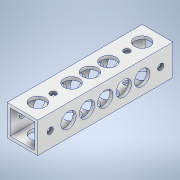
# Autodesk Inventor part: 前後直動12x12_3
Saved by Autodesk Inventor 2020.3 (Build 243373000, 373)
## iProperties
Created: 2020-07-05
Part Number: 前後直動12x12_3
Material: アルミニウム 6061
Document SubType Name: Modeling
Designer: totot
Density: 2.7 g/cm^3
Appearance: アルミニウム - フラット
Mass: 14.2052 g
Surface Area: 72.9 cm^2
Volume: 5.26118 cm^3
Author: totot
Autodesk Inventor part; units mm, degrees
ref_plane "YZ Plane" through (0, 0, 0) normal (1, 0, 0) x (0, 1, 0)
ref_plane "XZ Plane" through (0, 0, 0) normal (0, 1, 0) x (-1, 0, 0)
ref_plane "XY Plane" through (0, 0, 0) normal (0, 0, 1) x (1, 0, 0)
sketch "スケッチ1" plane through (0, 0, 0) normal (0, 0, 1) x (1, 0, 0)
  line L0 (0, 0) -> (-15, 0)
  line L1 (-15, 0) -> (-15, -15)
  line L2 (-15, -15) -> (0, -15)
  line L3 (0, -15) -> (0, 0)
  line L4 (-13.5, -1.5) -> (-1.5, -1.5)
  line L5 (-1.5, -1.5) -> (-1.5, -13.5)
  line L6 (-1.5, -13.5) -> (-13.5, -13.5)
  line L7 (-13.5, -13.5) -> (-13.5, -1.5)
  dimension "d0" = 15
  dimension "d1" = 15
  dimension "d2" = 12
  dimension "d3" = 12
  dimension "d4" = 1.5
  dimension "d5" = 1.5
  constraints: 16 end point, 4 parallel, 2 horizontal, 2 perpendicular
  measures "d0" distance of L2.end L1.end
  measures "d1" distance of L1.end L0.end
  measures "d2" distance of L5.end L6.end
  measures "d3" distance of L4.end L5.end
  measures "d4" distance between parallel lines of L1 L7
  measures "d5" distance between parallel lines of L4 L0
extrude "押し出し1" add sketch "スケッチ1" along normal blind 66
sketch "スケッチ2" plane through (0, -15, 0) normal (1, 0, 0) x (0, 0, -1)
  line L0 (0, 15) -> (-66, 15) projected
  line L1 (0, 0) -> (0, 15) projected
  line L2 (-66, 0) -> (-66, 15) projected
  point P0 (-60, 7.5)
  point P1 (-6, 7.5)
  dimension "d8" = 7.5
  dimension "d9" = 7.5
  dimension "d10" = 6
  dimension "d11" = 6
  measures "d8" distance from line of point (-60, 7.5) L0
  measures "d9" distance from line of point (-6, 7.5) L0
  measures "d10" distance from line of point (-6, 7.5) L1
  measures "d11" distance from line of point (-60, 7.5) L2
hole "穴1" at (0, -7.5, 60) at (0, -7.5, 6) direction (-1, 0, 0) diameter 3 end through all
sketch "スケッチ3" plane through (-15, -15, 0) normal (0, -1, 0) x (1, 0, 0)
  line L0 (0, 0) -> (0, 66) projected
  line L1 (0, 66) -> (15, 66) projected
  line L2 (0, 0) -> (15, 0) projected
  point P0 (7.5, 51)
  point P1 (7.5, 15)
  dimension "d19" = 7.5
  dimension "d20" = 7.5
  dimension "d21" = 15
  dimension "d22" = 15
  measures "d19" distance from line of L0 point (7.5, 51)
  measures "d20" distance from line of L0 point (7.5, 15)
  measures "d21" distance from line of point (7.5, 51) L1
  measures "d22" distance from line of L2 point (7.5, 15)
hole "穴2" at (-7.5, -15, 51) at (-7.5, -15, 15) direction (0, 1, 0) diameter 3 end through all
sketch "スケッチ4" plane through (-15, 0, 0) normal (0, 1, 0) x (1, 0, 0)
  line L0 (15, 0) -> (0, 0) projected
  line L1 (0, 0) -> (0, -66) projected
  line L2 (15, -66) -> (0, -66) projected
  circle A0 centre (7.5, -51) radius 1.5 projected
  circle A1 centre (7.5, -15) radius 1.5 projected
  point P0 (7.5, -7.5)
  point P1 (7.5, -58.5)
  point P2 (7.5, -42)
  point P3 (7.5, -33)
  point P4 (7.5, -24)
  dimension "d30" = 7.5
  dimension "d31" = 7.5
  dimension "d32" = 7.5
  dimension "d33" = 7.5
  dimension "d34" = 7.5
  dimension "d35" = 7.5
  dimension "d36" = 36
  dimension "d37" = 7.5
  dimension "d38" = 9
  dimension "d39" = 9
  dimension "d40" = 9
  measures "d30" distance from line of point (7.5, -7.5) L0
  measures "d31" distance from line of point (7.5, -7.5) L1
  measures "d32" distance from line of L2 point (7.5, -58.5)
  measures "d33" distance from line of L1 point (7.5, -58.5)
  measures "d34" distance from line of L1 point (7.5, -33)
  measures "d35" distance from line of L1 point (7.5, -42)
  measures "d36" distance of A0.centre A1.centre
  measures "d37" distance from line of L1 point (7.5, -24)
  measures "d38" distance of point (7.5, -24) A1.centre
  measures "d39" distance of A0.centre point (7.5, -42)
  measures "d40" distance of point (7.5, -42) point (7.5, -33)
hole "穴3" at (-7.5, 0, 7.5) at (-7.5, 0, 58.5) at (-7.5, 0, 42) at (-7.5, 0, 33) at (-7.5, 0, 24) direction (0, -1, 0) diameter 7.5 end through all
sketch "スケッチ5" plane through (0, -15, 0) normal (1, 0, 0) x (0, 0, -1)
  circle A0 centre (-60, 7.5) radius 1.5 projected
  circle A1 centre (-6, 7.5) radius 1.5 projected
  line L0 (-60, 7.5) -> (-6, 7.5)
  point P0 (0, 15)
  point P1 (-51, 7.5)
  point P2 (-42, 7.5)
  point P3 (-33, 7.5)
  point P4 (-24, 7.5)
  point P5 (-15, 7.5)
  dimension "d48" = 54
  dimension "d51" = 9
  dimension "d56" = 9
  constraints: 2 end point, 2 horizontal, 1 point on line, 4 other
  measures "d48" distance of L0.end L0.start
  measures "d51" distance of point (-51, 7.5) point (-42, 7.5)
  measures "d56" distance of L0.start point (-51, 7.5)
hole "穴4" at (0, -7.5, 51) at (0, -7.5, 42) at (0, -7.5, 33) at (0, -7.5, 24) at (0, -7.5, 15) direction (-1, 0, 0) diameter 7.5 end through all
equation "\"d1\" = d0"
equation "\"d3\" = d2"
equation "\"d5\" = d4"
equation "\"d9\" = d8"
equation "\"d20\" = d19"
equation "\"d21\" = d22"
equation "\"d31\" = d30"
equation "\"d32\" = d30"
equation "\"d33\" = d32"
equation "\"d35\" = d34"
equation "\"d38\" = 0.25 * d36"
equation "\"d39\" = d38"
equation "\"d40\" = d39"
equation "\"d56\" = d51"
